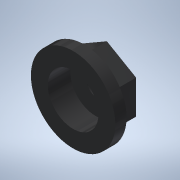
# Autodesk Inventor part: shocks_mover
Saved by Autodesk Inventor 2020 (Build 240168000, 168)
## iProperties
Created: 2015-12-04
Part Number: shocks_mover
Material: Goma
Document SubType Name: Modeling
Designer: MIGUEL ANGEL
Density: 0.93 g/cm^3
Appearance: Goma - Negro - Versión 1.1
Author: MIGUEL ANGEL
Autodesk Inventor part; units mm, degrees
ref_plane "YZ Plane" through (0, 0, 0) normal (1, 0, 0) x (0, 1, 0)
ref_plane "XZ Plane" through (0, 0, 0) normal (0, 1, 0) x (-1, 0, 0)
ref_plane "XY Plane" through (0, 0, 0) normal (0, 0, 1) x (1, 0, 0)
sketch "Boceto1" plane through (0, 0, 0) normal (0, 1, 0) x (-1, 0, 0)
  circle A0 centre (0, 0) radius 15
  dimension "d0" = 30
  constraints: 1 centre point, 1 coincident
  measures "d0" diameter of A0
extrude "Extrusión1" add sketch "Boceto1" along normal blind 4
sketch "Boceto2" plane through (0, 4, 0) normal (0, 1, 0) x (1, 0, 0)
  line L0 (10.3923, 6) -> (10.3923, -6)
  line L1 (10.3923, -6) -> (0, -12)
  line L2 (0, -12) -> (-10.3923, -6)
  line L3 (-10.3923, -6) -> (-10.3923, 6)
  line L4 (-10.3923, 6) -> (0, 12)
  line L5 (0, 12) -> (10.3923, 6)
  point P0 (0, 0)
  point P1 (0, 0)
  point P2 (10.3923, 0)
  dimension "d3" = 12
  constraints: 12 end point, 1 coincident, 1 horizontal alignment, 1 midpoint, 13 other
  measures "d3" distance of L0.start L0.end
extrude "Extrusión2" add sketch "Boceto2" along normal blind 8
sketch "Boceto3" plane through (0, 0, 0) normal (0, -1, 0) x (1, 0, 0)
  circle A0 centre (0, 0) radius 9
  dimension "d6" = 18
  constraints: 1 centre point, 1 coincident
  measures "d6" diameter of A0
extrude "Extrusión3" cut sketch "Boceto3" against normal blind 8
sketch "Boceto4" plane through (0, 12, 0) normal (0, 1, 0) x (1, 0, 0)
  circle A0 centre (0, 0) radius 3
  dimension "d9" = 6
  constraints: 1 centre point, 1 coincident
  measures "d9" diameter of A0
extrude "Extrusión4" cut sketch "Boceto4" against normal up to next
